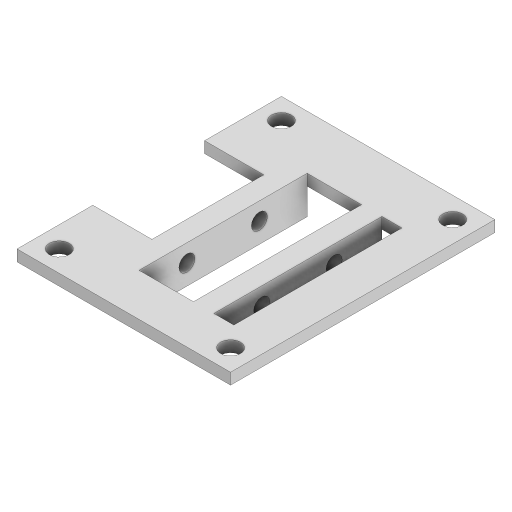
# Autodesk Inventor part: Scanner_Test_Top
Saved by Autodesk Inventor 2023 (Build 270158000, 158)
## iProperties
Created: 2022-09-22
Part Number: Scanner_Test_Top
Material: Generic
Document SubType Name: Modeling
Designer: Vking
Density: 1 g/cm^3
Appearance: Default
Author: Vking
Autodesk Inventor part; units mm, degrees
ref_plane "YZ Plane" through (0, 0, 0) normal (1, 0, 0) x (0, 1, 0)
ref_plane "XZ Plane" through (0, 0, 0) normal (0, 1, 0) x (-1, 0, 0)
ref_plane "XY Plane" through (0, 0, 0) normal (0, 0, 1) x (1, 0, 0)
sketch "Sketch1" plane through (0, 0, 0) normal (0, 0, 1) x (1, 0, 0)
  line L0 (-31.75, 5.08) -> (31.75, 5.08)
  line L1 (31.75, 5.08) -> (31.75, -5.08)
  line L2 (31.75, -5.08) -> (-31.75, -5.08)
  line L3 (-31.75, -5.08) -> (-31.75, 5.08)
  point P0 (0, 0)
  dimension "d0" = 63.5
  dimension "d3" = 31.75
  dimension "d4" = 10.16
  dimension "d17" = 5.08
  constraints: 8 end point, 2 parallel, 1 horizontal, 1 perpendicular
  measures "d0" distance of L0.start L0.end
  measures "d3" distance from line of L3 point (0, 0)
  measures "d4" distance of L0.end L1.end
  measures "d17" distance from line of point (0, 0) L2
extrude "Extrusion1" add sketch "Sketch1" along normal blind 76.2
sketch "Sketch9" plane through (-31.75, 5.08, 0) normal (0, 1, 0) x (1, 0, 0)
  line L0 (28.35, -18.7333) -> (35.15, -18.7333)
  line L1 (35.15, -18.7333) -> (35.15, -39.7333)
  line L2 (35.15, -39.7333) -> (28.35, -39.7333)
  line L3 (28.35, -39.7333) -> (28.35, -18.7333)
  line L4 (0, 0) -> (0, -76.2) projected
  line L5 (63.5, 0) -> (0, 0) projected
  point P0 (31.75, 0)
  point P1 (0, -38.1)
  dimension "d31" = 21
  dimension "d32" = 6.8
  dimension "d33" = 28.35
  dimension "d34" = 18.7333
  constraints: 8 end point, 2 parallel, 1 horizontal, 1 midpoint, 1 perpendicular
  measures "d31" distance of L0.end L1.end
  measures "d32" distance of L1.end L2.end
  measures "d33" distance from line of point (0, -38.1) L3
  measures "d34" distance between parallel lines of L0 L5
extrude "Extrusion8" cut sketch "Sketch9" against normal blind 19.5
sketch "Sketch28" plane through (-31.75, -5.08, 0) normal (0, -1, 0) x (1, 0, 0)
  line L0 (51.7099, 9.6993) -> (7.0225, 9.6993)
  line L1 (51.7099, 55.2865) -> (51.7099, 9.6993)
  line L2 (44.4458, 44.405) -> (19.0458, 44.405)
  line L3 (19.0458, 44.405) -> (19.0458, 12.655)
  line L4 (19.0458, 12.655) -> (44.4458, 12.655)
  line L5 (44.4458, 12.655) -> (44.4458, 44.405)
  line L6 (23.85, 39.7333) -> (30.65, 39.7333)
  line L7 (41.4458, 41.405) -> (22.0458, 41.405)
  line L8 (22.0458, 41.405) -> (22.0458, 15.655)
  line L9 (22.0458, 15.655) -> (41.4458, 15.655)
  line L10 (41.4458, 15.655) -> (41.4458, 41.405)
  circle A0 centre (42.4458, 42.405) radius 1.25
  circle A1 centre (42.4458, 14.655) radius 1.25
  circle A2 centre (21.0458, 14.655) radius 1.25
  circle A3 centre (21.0458, 42.405) radius 1.25
  line L11 (35.15, 39.7333) -> (35.15, 18.7333)
  line L12 (35.15, 18.7333) -> (28.35, 18.7333)
  line L13 (28.35, 18.7333) -> (28.35, 39.7333)
  line L14 (28.35, 39.7333) -> (35.15, 39.7333)
  line L15 (35.15, 39.7333) -> (35.15, 18.7333) projected
  line L16 (63.5, 0) -> (63.5, 76.2) projected
  line L17 (0, 76.2) -> (63.5, 76.2) projected
  line L18 (63.5, 0) -> (0, 0)
  line L19 (0, 0) -> (0, 76.2)
  line L20 (0, 76.2) -> (63.5, 76.2)
  line L21 (63.5, 76.2) -> (63.5, 0)
  point P0 (31.75, 0)
  point P1 (31.7458, 15.655)
  dimension "d175" = 31.75
  dimension "d176" = 25.4
  dimension "d177" = 3
  dimension "d178" = 3
  dimension "d179" = 3
  dimension "d180" = 3
  dimension "d181" = 2.5
  dimension "d182" = 2
  dimension "d183" = 2
  dimension "d184" = 2.5
  dimension "d185" = 2.5
  dimension "d186" = 2.5
  dimension "d188" = 2
  dimension "d190" = 2
  dimension "d191" = 2
  dimension "d192" = 2
  dimension "d193" = 0
  dimension "d194" = 6.8
  dimension "d195" = 21
  dimension "d196" = 6.2958
  dimension "d197" = 3.0783
  dimension "d268" = 2
  dimension "d269" = 2
  constraints: 38 end point, 6 parallel, 4 centre point, 4 horizontal, 3 perpendicular, 1 midpoint
  measures "d175" distance of L5.start L5.end
  measures "d176" distance of L4.start L5.start
  measures "d177" distance between parallel lines of L2 L7
  measures "d178" distance between parallel lines of L10 L5
  measures "d179" distance between parallel lines of L9 L4
  measures "d180" distance between parallel lines of L3 L8
  measures "d181" diameter of A0
  measures "d182" distance from line of L2 A0.centre
  measures "d183" distance from line of A0.centre L5
  measures "d184" diameter of A1
  measures "d185" diameter of A2
  measures "d186" diameter of A3
  measures "d188" distance from line of L2 A3.centre
  measures "d190" distance from line of L4 A2.centre
  measures "d191" distance from line of L5 A1.centre
  measures "d192" distance from line of A1.centre L4
  measures "d193" distance between parallel lines of L15 L11
  measures "d194" distance of L12.start L12.end
  measures "d195" distance of L12.end L14.start
  measures "d196" distance between parallel lines of L11 L10
  measures "d197" distance from line of L12 point (31.746, 15.655)
  measures "d268" distance from line of L3 A2.centre
  measures "d269" distance from line of L3 A3.centre
extrude "Extrusion18" cut sketch "Sketch28" against normal blind 25.4 contours L18 L19 L17 L16
extrude "Extrusion19" cut sketch "Sketch28" against normal blind 25.4 contours A0 | A1 | A2 | A3
sketch "Sketch29" plane through (-12.7042, -5.08, 12.655) normal (-1, 0, 0) x (0, 0, 1)
  line L0 (0, 10.16) -> (31.75, 10.16) projected
  line L1 (0, 0) -> (0, 10.16) projected
  line L2 (31.75, 0) -> (0, 0) projected
  line L3 (31.75, 0) -> (31.75, 10.16) projected
  line L4 (31.75, 0) -> (31.75, 10.16) projected
  line L5 (31.75, 0) -> (0, 0)
  line L6 (0, 0) -> (0, 1)
  line L7 (0, 1) -> (31.75, 1)
  line L8 (31.75, 1) -> (31.75, 0)
  line L9 (31.75, 1) -> (0, 1)
  line L10 (0, 1) -> (0, 10.16)
  line L11 (0, 10.16) -> (31.75, 10.16)
  line L12 (31.75, 10.16) -> (31.75, 1)
  point P0 (-12.655, 5.08)
  point P1 (31.75, 1)
  dimension "d202" = 1
  constraints: 16 end point, 4 parallel, 2 horizontal, 2 perpendicular, 1 point on line
  measures "d202" distance between parallel lines of L7 L2
extrude "Extrusion20" cut sketch "Sketch29" against normal blind 25.4 contours L0 L3 L7 L1
sketch "Sketch30" plane through (-12.7042, -4.08, 44.405) normal (0, 1, 0) x (1, 0, 0)
  line L0 (9.3042, 25.6717) -> (9.3042, 4.6717) projected
  circle A0 centre (2, 29.75) radius 1.25 projected
  circle A1 centre (23.4, 29.75) radius 1.25 projected
  circle A2 centre (2, 2) radius 1.25 projected
  circle A3 centre (23.4, 2) radius 1.25 projected
  line L1 (9.3042, 25.6717) -> (9.3042, 4.6717) projected
  line L2 (16.1042, 25.6717) -> (9.3042, 25.6717) projected
  line L3 (16.1042, 4.6717) -> (16.1042, 25.6717) projected
  line L4 (9.3042, 4.6717) -> (16.1042, 4.6717) projected
  line L5 (0, 0) -> (0, 31.75) projected
  line L6 (25.4, 0) -> (0, 0) projected
  line L7 (25.4, 31.75) -> (25.4, 0) projected
  line L8 (0, 31.75) -> (25.4, 31.75) projected
  line L9 (9.3042, 4.6717) -> (16.1042, 4.6717) projected
  line L10 (9.3042, 4.6717) -> (6.7642, 4.6717)
  line L11 (6.7642, 4.6717) -> (6.7642, 25.6717)
  line L12 (6.7642, 25.6717) -> (9.3042, 25.6717)
  line L13 (9.3042, 25.6717) -> (9.3042, 4.6717)
  line L14 (16.1042, 4.6717) -> (18.6442, 4.6717)
  line L15 (18.6442, 4.6717) -> (18.6442, 25.6717)
  line L16 (18.6442, 25.6717) -> (16.1042, 25.6717)
  line L17 (16.1042, 25.6717) -> (16.1042, 4.6717)
  point P0 (12.7042, 44.405)
  point P1 (9.3042, 25.6717)
  dimension "d205" = 2.54
  dimension "d206" = 2.54
  constraints: 16 end point, 4 parallel, 2 horizontal, 2 perpendicular, 1 point on line
  measures "d205" distance between parallel lines of L0 L11
  measures "d206" distance between parallel lines of L17 L15
extrude "Extrusion21" add sketch "Sketch30" along normal blind 3.699 contours L0 L10 L11 L12 | L16 L15 L14 L3
sketch "Sketch31" plane through (-5.94, -4.08, 18.7333) normal (-1, 0, 0) x (0, 0, 1)
  circle A0 centre (15.0216, 1.199) radius 1
  circle A1 centre (5.9726, 1.199) radius 1
  line L0 (0, 3.699) -> (21, 3.699) projected
  line L1 (21, 0) -> (21, 3.699) projected
  line L2 (0, 0) -> (0, 3.699) projected
  line L3 (16.0216, 0.199) -> (4.9726, 0.199)
  line L4 (4.9726, 0.199) -> (4.9726, 2.199)
  line L5 (4.9726, 2.199) -> (16.0216, 2.199)
  line L6 (16.0216, 2.199) -> (16.0216, 0.199)
  point P0 (-18.7333, 4.08)
  point P1 (21, 1.8495)
  dimension "d209" = 2
  dimension "d210" = 2
  dimension "d213" = 2.5
  dimension "d214" = 2.5
  dimension "d227" = 11.049
  dimension "d228" = 21
  dimension "d229" = 4.9784
  constraints: 8 end point, 4 tangent, 2 centre point, 2 parallel, 1 horizontal, 1 midpoint, 1 perpendicular
  measures "d209" diameter of A1
  measures "d210" diameter of A0
  measures "d213" distance from line of L0 A1.centre
  measures "d214" distance from line of L0 A0.centre
  measures "d227" distance of L3.start L3.end
  measures "d228" distance of L0.start L0.end
  measures "d229" distance between parallel lines of L1 L6
extrude "Extrusion22" cut sketch "Sketch31" against normal blind 25.4 contours A0 | A1
sketch "Sketch32" plane through (-12.7042, -4.08, 44.405) normal (0, 1, 0) x (1, 0, 0)
  line L0 (18.6442, 4.6717) -> (16.1042, 4.6717) projected
  line L1 (9.3042, 4.6717) -> (16.1042, 4.6717) projected
  line L2 (9.3042, 4.6717) -> (6.7642, 4.6717) projected
  line L3 (6.7642, 4.6717) -> (6.7642, 25.6717) projected
  line L4 (6.7642, 25.6717) -> (9.3042, 25.6717) projected
  line L5 (16.1042, 25.6717) -> (9.3042, 25.6717) projected
  line L6 (16.1042, 25.6717) -> (18.6442, 25.6717) projected
  line L7 (18.6442, 25.6717) -> (18.6442, 4.6717) projected
  circle A0 centre (2, 29.75) radius 1.25 projected
  circle A1 centre (23.4, 29.75) radius 1.25 projected
  circle A2 centre (2, 2) radius 1.25 projected
  circle A3 centre (23.4, 2) radius 1.25 projected
  line L8 (0, 0) -> (0, 31.75) projected
  line L9 (25.4, 0) -> (0, 0) projected
  line L10 (25.4, 31.75) -> (25.4, 0) projected
  line L11 (0, 31.75) -> (25.4, 31.75) projected
  line L12 (6.7642, 25.6717) -> (4.2642, 25.6717)
  line L13 (4.2642, 25.6717) -> (4.2642, 4.6717)
  line L14 (4.2642, 4.6717) -> (6.7642, 4.6717)
  line L15 (6.7642, 4.6717) -> (6.7642, 25.6717)
  line L16 (18.6442, 25.6717) -> (21.1442, 25.6717)
  line L17 (21.1442, 25.6717) -> (21.1442, 4.6717)
  line L18 (21.1442, 4.6717) -> (18.6442, 4.6717)
  line L19 (18.6442, 4.6717) -> (18.6442, 25.6717)
  line L20 (6.7642, 12.6346) -> (4.2642, 12.6346)
  line L21 (4.2642, 12.6346) -> (4.2642, 18.9846)
  line L22 (4.2642, 18.9846) -> (6.7642, 18.9846)
  line L23 (6.7642, 18.9846) -> (6.7642, 12.6346)
  line L24 (18.6442, 12.6346) -> (21.1442, 12.6346)
  line L25 (21.1442, 12.6346) -> (21.1442, 18.9846)
  line L26 (21.1442, 18.9846) -> (18.6442, 18.9846)
  line L27 (18.6442, 18.9846) -> (18.6442, 12.6346)
  point P0 (12.7042, 44.405)
  point P1 (6.7642, 4.6717)
  point P2 (19.8942, 12.6346)
  point P3 (6.7642, 12.6346)
  point P4 (4.2642, 12.6346)
  point P5 (6.7642, 18.9846)
  point P6 (18.6442, 18.9846)
  point P7 (5.5142, 18.9846)
  dimension "d217" = 2.5
  dimension "d218" = 2.5
  dimension "d221" = 6.35
  dimension "d222" = 21
  dimension "d223" = 7.9629
  constraints: 32 end point, 8 parallel, 7 point on line, 4 horizontal, 4 perpendicular, 2 midpoint
  measures "d217" distance between parallel lines of L15 L13
  measures "d218" distance between parallel lines of L19 L17
  measures "d221" distance from line of point (19.894, 12.635) L26
  measures "d222" distance of L12.end L13.end
  measures "d223" distance between parallel lines of L18 L24
extrude "Extrusion23" cut sketch "Sketch32" against normal blind 25.4 contours L7 L24 L17 L18 | L7 L16 L17 L26 | L14 L13 L20 L3 | L22 L13 L12 L3
sketch "Sketch33" plane through (-12.7042, -5.08, 12.655) normal (0, -1, 0) x (1, 0, 0)
  line L0 (16.1042, 11.0509) -> (18.6442, 11.0509) projected
  line L1 (16.1042, 13.0509) -> (18.6442, 13.0509) projected
  line L2 (16.1042, 20.0999) -> (16.1042, 22.0999) projected
  line L3 (16.1042, 20.0999) -> (18.6442, 20.0999) projected
  line L4 (16.1042, 22.0999) -> (18.6442, 22.0999) projected
  line L5 (21.1442, 6.0783) -> (21.1442, 12.7654) projected
  line L6 (25.4, 0) -> (25.4, 31.75) projected
  line L7 (18.6442, 8.9554) -> (25.4, 8.9554)
  line L8 (25.4, 8.9554) -> (25.4, 14.0354)
  line L9 (25.4, 14.0354) -> (18.6442, 14.0354)
  line L10 (18.6442, 14.0354) -> (18.6442, 8.9554)
  line L11 (21.1442, 27.0783) -> (21.1442, 19.1154) projected
  line L12 (18.6442, 17.8454) -> (25.4, 17.8454)
  line L13 (25.4, 17.8454) -> (25.4, 22.9254)
  line L14 (25.4, 22.9254) -> (18.6442, 22.9254)
  line L15 (18.6442, 22.9254) -> (18.6442, 17.8454)
  line L16 (18.6442, 12.7654) -> (21.1442, 12.7654) projected
  line L17 (21.1442, 19.1154) -> (18.6442, 19.1154) projected
  line L18 (18.6442, 19.1154) -> (18.6442, 27.0783) projected
  line L19 (18.6442, 6.0783) -> (18.6442, 12.7654) projected
  point P0 (12.7042, -12.655)
  point P1 (21.1442, 22.9254)
  point P2 (20.8442, 13.4004)
  point P3 (25.4, 8.9554)
  point P4 (19.8942, 12.7654)
  point P5 (20.8442, 13.4004)
  point P6 (18.6442, 12.7654)
  point P7 (21.1442, 8.9554)
  point P8 (18.6442, 8.9554)
  dimension "d235" = 5.08
  dimension "d236" = 3.81
  dimension "d237" = 1.27
  dimension "d239" = 1.27
  dimension "d240" = 0
  dimension "d241" = 0
  constraints: 16 end point, 3 parallel, 2 horizontal, 2 perpendicular, 2 point on line, 1 midpoint
  measures "d235" distance between parallel lines of L14 L12
  measures "d236" distance between parallel lines of L16 L7
  measures "d237" distance from line of point (19.894, 12.765) L9
  measures "d239" distance between parallel lines of L17 L12
  measures "d240" distance between parallel lines of L18 L15
  measures "d241" distance between parallel lines of L19 L10
extrude "Extrusion24" cut sketch "Sketch33" against normal blind 25.4 contours L6 L7 L5 L16 L10 L9 | L15 L14 L11 L17 | L17 L11 L14 L6 L12 L15 | L7 L10 L16 L5
sketch "Sketch36" plane through (-12.7042, -5.08, 44.405) normal (0, -1, 0) x (1, 0, 0)
  line L0 (18.6442, -17.7146) -> (25.4, -17.7146) projected
  line L1 (25.4, -13.9046) -> (18.6442, -13.9046) projected
  line L2 (18.6442, -17.7146) -> (25.4, -17.7146)
  line L3 (25.4, -17.7146) -> (25.4, -13.9046)
  line L4 (25.4, -13.9046) -> (18.6442, -13.9046)
  line L5 (18.6442, -13.9046) -> (18.6442, -17.7146)
  point P0 (12.7042, -44.405)
  constraints: 8 end point, 2 parallel, 1 horizontal, 1 perpendicular
extrude "Extrusion26" cut sketch "Sketch36" against normal blind 1
sketch "Sketch37" plane through (-12.7042, -5.08, 44.405) normal (0, -1, 0) x (1, 0, 0)
  line L0 (25.4, -8.8246) -> (25.4, 0) projected
  line L1 (0, -31.75) -> (25.4, -31.75) projected
  line L2 (25.4, 0) -> (0, 0)
  line L3 (0, 0) -> (0, -31.75)
  line L4 (0, -31.75) -> (25.4, -31.75)
  line L5 (25.4, -31.75) -> (25.4, 0)
  line L6 (26.035, 0.635) -> (-0.635, 0.635)
  line L7 (-0.635, 0.635) -> (-0.635, -32.385)
  line L8 (-0.635, -32.385) -> (26.035, -32.385)
  line L9 (26.035, -32.385) -> (26.035, 0.635)
  line L10 (26.035, -8.8246) -> (25.4, -8.8246)
  line L11 (18.6442, -22.1596) -> (25.4, -22.1596) projected
  line L12 (25.4, -22.7946) -> (26.035, -22.7946)
  point P0 (12.7042, -44.405)
  dimension "d247" = 0.635
  constraints: 20 end point, 4 parallel, 3 perpendicular, 2 horizontal, 2 point on line, 3 other
  measures "d247" distance between parallel lines of L5 L9
extrude "Extrusion27" add sketch "Sketch37" against normal blind 1 contours L0 L2 L3 L1 L5 L12 L9 L8 L7 L6 L10
sketch "Sketch39" plane through (-3.4, -4.08, 39.7333) normal (0, 1, 0) x (1, 0, 0)
  line L0 (9.34, 0) -> (6.8, 0) projected
  line L1 (0, 0) -> (6.8, 0) projected
  line L2 (0, 0) -> (-2.54, 0) projected
  line L3 (-2.54, 0) -> (-5.04, 0) projected
  line L4 (-5.04, 0) -> (-5.04, 7.9629) projected
  line L5 (-5.04, 7.9629) -> (-2.54, 7.9629) projected
  line L6 (-2.54, 7.9629) -> (-2.54, 14.3129) projected
  line L7 (-2.54, 14.3129) -> (-5.04, 14.3129) projected
  line L8 (-5.04, 14.3129) -> (-5.04, 21) projected
  line L9 (-5.04, 21) -> (-2.54, 21) projected
  line L10 (-2.54, 21) -> (0, 21) projected
  line L11 (6.8, 21) -> (0, 21) projected
  line L12 (6.8, 21) -> (9.34, 21) projected
  line L13 (16.7308, 18.1229) -> (16.7308, 27.7133) projected
  line L14 (16.7308, 27.7133) -> (-9.9392, 27.7133) projected
  line L15 (-9.9392, 27.7133) -> (-9.9392, -5.3067) projected
  line L16 (-9.9392, -5.3067) -> (16.7308, -5.3067) projected
  line L17 (16.7308, -5.3067) -> (16.7308, 4.1529) projected
  circle A0 centre (-7.3042, 25.0783) radius 1.25 projected
  circle A1 centre (14.0958, 25.0783) radius 1.25 projected
  circle A2 centre (-7.3042, -2.6717) radius 1.25 projected
  circle A3 centre (14.0958, -2.6717) radius 1.25 projected
  line L18 (16.7308, 4.1529) -> (11.84, 4.1529) projected
  line L19 (11.84, 4.1529) -> (11.84, 0) projected
  line L20 (9.34, 21) -> (11.84, 21) projected
  line L21 (11.84, 21) -> (11.84, 18.1229) projected
  line L22 (11.84, 18.1229) -> (16.7308, 18.1229) projected
  line L23 (9.34, 0) -> (9.34, 21) projected
  line L24 (11.84, 3.5179) -> (9.34, 3.5179)
  line L25 (9.34, 3.5179) -> (9.34, 0)
  line L26 (9.34, 0) -> (11.84, 0)
  line L27 (11.84, 0) -> (11.84, 3.5179)
  line L28 (11.84, 0) -> (9.34, 0) projected
  point P0 (3.4, 39.7333)
  point P1 (9.34, 3.5179)
  constraints: 8 end point, 2 parallel, 1 horizontal, 1 perpendicular
extrude "Extrusion28" add sketch "Sketch39" along normal blind 0.4 contours L26 L19 L18 L17 L16 L15 L14 L13 L22 L21 L20 L12 L11 L10 L9 L8 L7 L6 L5 L4 L3 L2 L1 L0
sketch "Sketch40" plane through (5.94, -5.08, 18.7333) normal (0, -1, 0) x (1, 0, 0)
  line L0 (-14.38, 6.6871) -> (-11.88, 6.6871) projected
  line L1 (-11.88, 6.6871) -> (-11.88, 0) projected
  line L2 (-11.88, 0) -> (-14.38, 0) projected
  line L3 (-14.38, 0) -> (-14.38, 6.6871) projected
  line L4 (0, 0) -> (0, 21) projected
  line L5 (2.5, 21) -> (2.5, 16.8471) projected
  line L6 (2.5, 16.8471) -> (7.3908, 16.8471) projected
  line L7 (7.3908, 16.8471) -> (7.3908, 26.3067) projected
  line L8 (7.3908, 26.3067) -> (-19.2792, 26.3067) projected
  line L9 (-19.2792, 26.3067) -> (-19.2792, -6.7133) projected
  line L10 (-19.2792, -6.7133) -> (7.3908, -6.7133) projected
  line L11 (7.3908, -6.7133) -> (7.3908, 2.8771) projected
  line L12 (7.3908, 2.8771) -> (2.5, 2.8771) projected
  line L13 (2.5, 2.8771) -> (2.5, 0) projected
  line L14 (2.5, 0) -> (0, 0) projected
  line L15 (-11.88, 13.0371) -> (-14.38, 13.0371) projected
  line L16 (-14.38, 13.0371) -> (-14.38, 21) projected
  line L17 (-14.38, 21) -> (-11.88, 21) projected
  line L18 (-11.88, 21) -> (-11.88, 13.0371) projected
  circle A0 centre (-16.6442, -4.0783) radius 1.25 projected
  circle A1 centre (4.7558, -4.0783) radius 1.25 projected
  circle A2 centre (-16.6442, 23.6717) radius 1.25 projected
  circle A3 centre (4.7558, 23.6717) radius 1.25 projected
  line L19 (-2.54, 21) -> (-2.54, 0) projected
  line L20 (-2.54, 0) -> (-9.34, 0) projected
  line L21 (-9.34, 0) -> (-9.34, 21) projected
  line L22 (-9.34, 21) -> (-2.54, 21) projected
  line L23 (0, 21) -> (0, 0) projected
  line L24 (2.5, 17.4821) -> (0, 17.4821)
  line L25 (0, 17.4821) -> (0, 16.8471)
  line L26 (0, 16.8471) -> (2.5, 16.8471)
  line L27 (2.5, 16.8471) -> (2.5, 17.4821)
  line L28 (2.5, 2.8771) -> (0, 2.8771)
  line L29 (0, 2.8771) -> (0, 0)
  line L30 (0, 0) -> (2.5, 0)
  line L31 (2.5, 0) -> (2.5, 2.8771)
  line L32 (0, 21) -> (2.5, 21) projected
  point P0 (-5.94, -18.7333)
  point P1 (0, 17.4821)
  constraints: 16 end point, 4 parallel, 2 horizontal, 2 perpendicular, 1 point on line
extrude "Extrusion30" add sketch "Sketch40" against normal blind 1.4 contours L4 L28 L13 L14 | L4 L24 L5 L26 | L4 L32 L5 L24
sketch "Sketch41" plane through (5.94, -5.08, 21.6104) normal (0, -1, 0) x (1, 0, 0)
  line L0 (-11.88, 10.16) -> (-14.38, 10.16)
  line L1 (-14.38, 10.16) -> (-14.38, 3.81)
  line L2 (-14.38, 3.81) -> (-11.88, 3.81)
  line L3 (-11.88, 3.81) -> (-11.88, 10.16)
  point P0 (-5.94, -21.6104)
  constraints: 8 end point, 2 parallel, 1 horizontal, 1 perpendicular
extrude "Extrusion31" cut sketch "Sketch41" against normal blind 25.4
body "Solid1"
